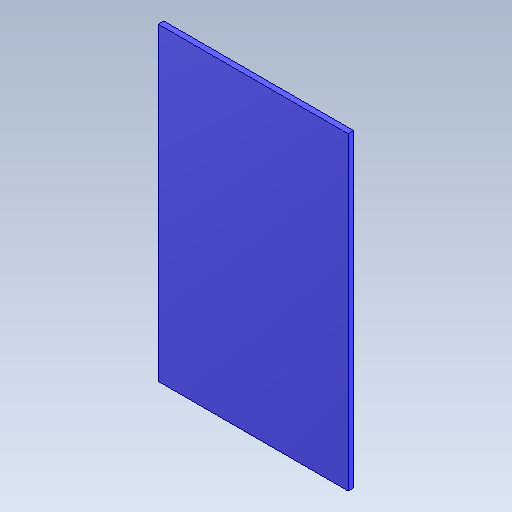
# Autodesk Inventor part: ST7735
Saved by Autodesk Inventor 2021 (Build 250183000, 183)
## iProperties
Created: 2020-11-03
Part Number: ST7735
Material: Generic
Document SubType Name: Modeling
Designer: faiya
Density: 1 g/cm^3
Appearance: ST7735, ST7735
Author: faiya
Autodesk Inventor part; units mm, degrees
ref_plane "YZ Plane" through (0, 0, 0) normal (1, 0, 0) x (0, 1, 0)
ref_plane "XZ Plane" through (0, 0, 0) normal (0, 1, 0) x (-1, 0, 0)
ref_plane "XY Plane" through (0, 0, 0) normal (0, 0, 1) x (1, 0, 0)
sketch "ST7735, ST7735_39" plane through (0, 0, 0) normal (0, 0, 1) x (1, 0, 0)
  line L0 (-15.9512, 22.9362) -> (18.415, 22.9362)
  line L1 (18.415, 22.9362) -> (18.415, -33.02)
  line L2 (18.415, -33.02) -> (-15.9512, -33.02)
  line L3 (-15.9512, -33.02) -> (-15.9512, 22.9362)
  constraints: 8 end point
extrude "Extrusion1" add sketch "ST7735, ST7735_39" along normal blind 1
body "Solid1"
